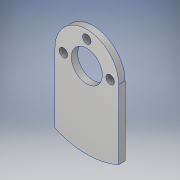
# Autodesk Inventor part: Gear Protection Piece
Saved by Autodesk Inventor 2019.4 (Build 234330000, 330)
## iProperties
Created: 2019-11-02
Part Number: Gear Protection Piece
Material: Aluminum 6061
Document SubType Name: Modeling
Designer: admin
Density: 2.7 g/cm^3
Appearance: Aluminum - Flat
Author: admin
Autodesk Inventor part; units mm, degrees
ref_plane "YZ Plane" through (0, 0, 0) normal (1, 0, 0) x (0, 1, 0)
ref_plane "XZ Plane" through (0, 0, 0) normal (0, 1, 0) x (-1, 0, 0)
ref_plane "XY Plane" through (0, 0, 0) normal (0, 0, 1) x (1, 0, 0)
sketch "Sketch1" plane through (0, 0, 0) normal (0, 0, 1) x (1, 0, 0)
  circle A0 centre (0, 0) radius 7.3
  arc A1 (-15, -32.7261) -> (15, -32.7261) centre (0, 0) ccw
  arc A2 (15, 0) -> (-15, 0) centre (0, 0) ccw
  line L0 (-15, 0) -> (-15, -32.7261)
  line L1 (15, 0) -> (15, -32.7261)
  arc A3 (15, -32.7261) -> (-15, -32.7261) centre (0, 0) ccw construction
  arc A4 (-15, 0) -> (15, 0) centre (0, 0) ccw construction
  dimension "d0" = 14.6
  dimension "d1" = 72
  dimension "d2" = 30
  constraints: 8 point on circle, 5 centre point, 4 end point, 3 coincident, 2 tangent, 1 parallel, 1 vertical
  measures "d0" diameter of A0
  measures "d1" diameter of A1
  measures "d2" diameter of A2
extrude "Extrusion1" add sketch "Sketch1" along normal blind 3
sketch "Sketch2" plane through (0, 0, 3) normal (0, 0, 1) x (1, 0, 0)
  circle A0 centre (-11, 0) radius 2
  circle A1 centre (11, 0) radius 2
  circle A2 centre (0, 11) radius 2
  line L0 (0, 0) -> (0, 11) construction
  line L1 (0, 0) -> (11, 0) construction
  line L2 (0, 0) -> (-11, 0) construction
  dimension "d5" = 4
  dimension "d6" = 4
  dimension "d7" = 4
  dimension "d8" = 11
  dimension "d9" = 11
  dimension "d10" = 11
  constraints: 6 end point, 3 centre point, 2 horizontal, 1 coincident, 1 vertical
  measures "d5" diameter of A0
  measures "d6" diameter of A1
  measures "d7" diameter of A2
  measures "d8" distance of L0.start L2.end
  measures "d9" distance of L0.start L1.end
  measures "d10" distance of L0.start L0.end
extrude "Extrusion2" cut sketch "Sketch2" against normal blind 3
body "Solid1"
